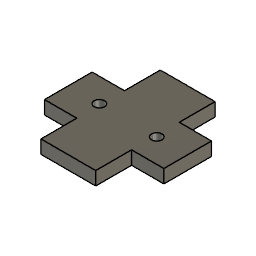
panel_bracket (Autodesk Fusion 360 design; units mm, degrees)
Autodesk Fusion 360 part; units mm, degrees
sketch "Sketch1" plane through (0, 0, 0) normal (0, 0, 1) x (1, 0, 0)
  line L0 (-9.18, -20) -> (9.18, -20)
  line L1 (9.18, -20) -> (9.18, 20)
  line L2 (9.18, 20) -> (-9.18, 20)
  line L3 (-9.18, 20) -> (-9.18, -20)
  circle A0 centre (9.6412, -0.0073) radius 1.75
  line L4 (-9.18, -7.9922) -> (-20, -7.9922)
  line L5 (-20, -7.9922) -> (-20, 8)
  line L6 (-20, 8) -> (-9.18, 8)
  line L7 (-9.18, 8) -> (-9.18, -7.9922)
  line L8 (20, -7.9922) -> (20, 8)
  line L9 (9.18, -7.9922) -> (20, -7.9922)
  line L10 (9.18, 8) -> (9.18, -7.9922)
  line L11 (20, 8) -> (9.18, 8)
  circle A1 centre (-9.5812, -0.0073) radius 1.75
  dimension "d1" = 18.36
  dimension "d2" = 40
  dimension "d3" = 3.5
  constraint horizontal L0
  constraint vertical L1
  constraint horizontal L2
  constraint vertical L3
  constraint horizontal L4
  constraint vertical L5
  constraint horizontal L6
  constraint vertical L7
  constraint coincident L3 L4.start
  measures "d1" distance of L0.start L0.end
  measures "d2" distance of L0.start L2.end
  measures "d3" diameter of A0
extrude "Extrude1" add sketch "Sketch1" along normal blind 4.5 makes body 1
extrude "Extrude2" cut sketch "Sketch1" along normal blind 5 contours L1 A0 L10 | L1 A0 L10 bodies 1
fillet "Fillet1" radius 1 12 edges at (9.18, -20, 2.25) (-9.18, -20, 2.25) (-20, -7.9922, 2.25) (-9.18, -7.9922, 2.25) (9.18, -7.9922, 2.25) (20, -7.9922, 2.25) (20, 8, 2.25) (9.18, 8, 2.25) (9.18, 20, 2.25) (-9.18, 20, 2.25) (-9.18, 8, 2.25) (-20, 8, 2.25) on bodies 1
extrude "Extrude3" add sketch "Sketch1" along normal blind 4.5 separate body makes body 2
extrude "Extrude4" cut sketch "Sketch1" along normal blind 5 contours L3 L7 A1 | L3 L7 A1 | L1 A0 L10 | L1 A0 L10 bodies 2
extrude "Extrude5" add sketch "Sketch1" along normal blind 4.5 separate body contours L0 L1 L2 L3 A0 L7 L10 A1 | L3 L4 L5 L6 L7 A1 | L1 A0 L8 L9 L10 L11 makes body 3
extrude "Extrude6" add sketch "Sketch1" along normal blind 4.5 separate body contours L0 L1 L2 L3 A0 L7 L10 A1 | L3 L4 L5 L6 L7 A1 | L1 A0 L8 L9 L10 L11 makes body 4
hidden bodies 1 2 3
